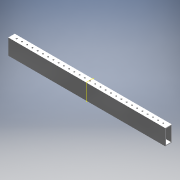
# Autodesk Inventor part: Front Extrusion
Saved by Autodesk Inventor 2019.4 (Build 234330000, 330)
## iProperties
Created: 2019-12-11
Part Number: Front Extrusion
Material: Aluminum 6061
Document SubType Name: Modeling
Designer: Mark
Mass: 882.774 g
Surface Area: 2224.42 cm^2
Volume: 326.953 cm^3
Density: 2.7 g/cm^3
Appearance: Aluminum - Flat
Author: Mark
Autodesk Inventor part; units mm, degrees
ref_plane "YZ Plane" through (0, 0, 0) normal (1, 0, 0) x (0, 1, 0)
ref_plane "XZ Plane" through (0, 0, 0) normal (0, 1, 0) x (-1, 0, 0)
ref_plane "XY Plane" through (0, 0, 0) normal (0, 0, 1) x (1, 0, 0)
sketch "Sketch1" plane through (0, 0, 0) normal (1, 0, 0) x (0, 1, 0)
  line L0 (-30, 12.5) -> (30, 12.5)
  line L1 (30, 12.5) -> (30, -12.5)
  line L2 (30, -12.5) -> (-30, -12.5)
  line L3 (-30, -12.5) -> (-30, 12.5)
  line L4 (-30, 12.5) -> (30, -12.5) construction
  line L5 (30, 12.5) -> (-30, -12.5) construction
  line L6 (-27, 9.5) -> (27, 9.5)
  line L7 (27, 9.5) -> (27, -9.5)
  line L8 (27, -9.5) -> (-27, -9.5)
  line L9 (-27, -9.5) -> (-27, 9.5)
  line L10 (-27, 9.5) -> (27, -9.5) construction
  line L11 (27, 9.5) -> (-27, -9.5) construction
  point P0 (0, 0)
  dimension "d0" = 60
  dimension "d1" = 25
  dimension "d2" = 54
  dimension "d3" = 19
  constraints: 24 end point, 4 midpoint, 4 parallel, 2 horizontal, 2 perpendicular
  measures "d0" distance of L1.end L2.end
  measures "d1" distance of L0.end L1.end
  measures "d2" distance of L7.end L8.end
  measures "d3" distance of L6.end L7.end
extrude "Extrusion1" add sketch "Sketch1" along normal blind 600
ref_plane "Work Plane1" through (300, 0, 0) normal (1, 0, 0) x (0, 0, -1)
sketch "Sketch2" plane through (0, 30, 12.5) normal (0, 1, 0) x (1, 0, 0)
  circle A0 centre (20, 12.5) radius 2.75
  line L0 (0, 0) -> (0, 25) projected
  line L1 (0, 0) -> (600, 0) projected
  circle A1 centre (40, 12.5) radius 2.75
  circle A2 centre (60, 12.5) radius 2.75
  circle A3 centre (80, 12.5) radius 2.75
  circle A4 centre (100, 12.5) radius 2.75
  circle A5 centre (120, 12.5) radius 2.75
  circle A6 centre (140, 12.5) radius 2.75
  circle A7 centre (160, 12.5) radius 2.75
  circle A8 centre (180, 12.5) radius 2.75
  circle A9 centre (200, 12.5) radius 2.75
  circle A10 centre (220, 12.5) radius 2.75
  circle A11 centre (240, 12.5) radius 2.75
  circle A12 centre (260, 12.5) radius 2.75
  circle A13 centre (280, 12.5) radius 2.75
  circle A14 centre (300, 12.5) radius 2.75
  circle A15 centre (320, 12.5) radius 2.75
  circle A16 centre (340, 12.5) radius 2.75
  circle A17 centre (360, 12.5) radius 2.75
  circle A18 centre (380, 12.5) radius 2.75
  circle A19 centre (400, 12.5) radius 2.75
  circle A20 centre (420, 12.5) radius 2.75
  circle A21 centre (440, 12.5) radius 2.75
  circle A22 centre (460, 12.5) radius 2.75
  circle A23 centre (480, 12.5) radius 2.75
  circle A24 centre (500, 12.5) radius 2.75
  circle A25 centre (520, 12.5) radius 2.75
  circle A26 centre (540, 12.5) radius 2.75
  circle A27 centre (560, 12.5) radius 2.75
  circle A28 centre (580, 12.5) radius 2.75
  circle A29 centre (600, 12.5) radius 2.75
  circle A30 centre (620, 12.5) radius 2.75
  circle A31 centre (640, 12.5) radius 2.75
  circle A32 centre (660, 12.5) radius 2.75
  circle A33 centre (680, 12.5) radius 2.75
  circle A34 centre (700, 12.5) radius 2.75
  circle A35 centre (720, 12.5) radius 2.75
  circle A36 centre (740, 12.5) radius 2.75
  circle A37 centre (760, 12.5) radius 2.75
  circle A38 centre (780, 12.5) radius 2.75
  circle A39 centre (800, 12.5) radius 2.75
  circle A40 centre (820, 12.5) radius 2.75
  circle A41 centre (840, 12.5) radius 2.75
  circle A42 centre (860, 12.5) radius 2.75
  circle A43 centre (880, 12.5) radius 2.75
  circle A44 centre (900, 12.5) radius 2.75
  circle A45 centre (920, 12.5) radius 2.75
  circle A46 centre (940, 12.5) radius 2.75
  circle A47 centre (960, 12.5) radius 2.75
  circle A48 centre (980, 12.5) radius 2.75
  circle A49 centre (1000, 12.5) radius 2.75
  point P0 (0, 12.5)
  dimension "d7" = 5.5
  dimension "d8" = 20
  dimension "d9" = 12.5
  dimension "d12" = 20
  constraints: 50 centre point, 1 horizontal, 98 other
  measures "d7" diameter of A0
  measures "d8" distance from line of A0.centre L0
  measures "d9" distance from line of L1 A0.centre
  measures "d12" distance of A0.centre A1.centre
extrude "Extrusion2" cut sketch "Sketch2" against normal blind 100 contours A0 | A1 | A2 | A3 | A4 | A5 | A6 | A7 | A8 | A9 | A10 | A11 | A12 | A13 | A14 | A15 | A16 | A17 | A18 | A19 | A20 | A21 | A22 | A23 | A24 | A25 | A26 | A27 | A28
equation "\"d4\" = Width"
equation "\"Width\" = 600"
body "Solid1"
